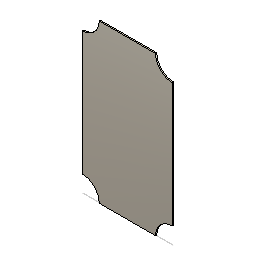
Base+Plate+2023 (Autodesk Fusion 360 design; units mm, degrees)
Autodesk Fusion 360 part; units mm, degrees
sketch "Sketch1" plane through (0, 0, 0) normal (0, 0, 1) x (1, 0, 0)
  line L0 (0, 0) -> (406.4, 0)
  line L1 (406.4, 0) -> (406.4, 711.2)
  line L2 (406.4, 711.2) -> (0, 711.2)
  line L3 (0, 711.2) -> (0, 0)
  arc A0 (0, 635) -> (76.2, 711.2) centre (0, 711.2) ccw
  arc A1 (330.2, 711.2) -> (406.4, 635) centre (406.4, 711.2) ccw
  arc A2 (76.2, 0) -> (0, 76.2) centre (0, 0) ccw
  arc A3 (406.4, 76.2) -> (330.2, 0) centre (406.4, 0) ccw
  dimension "d1" = 406.4
  dimension "d2" = 711.2
  dimension "d5" = 152.4
  dimension "d6" = 152.4
  dimension "d7" = 152.4
  dimension "d8" = 152.4
  constraint horizontal L0
  constraint vertical L1
  constraint horizontal L2
  constraint vertical L3
  constraint coincident L0.start L3.end
  constraint coincident L0.end L1.start
  constraint coincident L1.end L2.start
  constraint coincident L2.end L3.start
  constraint coincident L2 A0.end
  constraint coincident L3 A0.start
  constraint coincident L1 A1.end
  constraint coincident L2 A1.start
  constraint coincident L3 A2.end
  constraint coincident L0 A2.start
  constraint coincident L0 A3.end
  constraint coincident L1 A3.start
  measures "d1" distance of L0.start L0.end
  measures "d2" distance of L0.start L2.end
  measures "d5" diameter of A2
  measures "d6" diameter of A3
  measures "d7" diameter of A1
  measures "d8" diameter of A0
extrude "Extrude1" add sketch "Sketch1" along normal blind 5.715 contours L0 L1 L2 L3 A0 A1 A2 A3 makes body 1
copy_body "Body->Comp1" bodies 1 removing the originals makes body 2 in component "Component"
component "Component" placed x (1, 0, 0) y (0, 1, 0) z (0, 0, 1) at (0, 0, 0)
